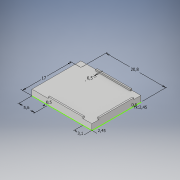
# Autodesk Inventor part: čip
Saved by Autodesk Inventor 2019 (Build 230136000, 136)
## iProperties
Created: 2020-07-28
Part Number: čip
Material: Generic
Document SubType Name: Modeling
Designer: lukad
Density: 1 g/cm^3
Appearance: Default
Author: lukad
Autodesk Inventor part; units mm, degrees
ref_plane "YZ Plane" through (0, 0, 0) normal (1, 0, 0) x (0, 1, 0)
ref_plane "XZ Plane" through (0, 0, 0) normal (0, 1, 0) x (-1, 0, 0)
ref_plane "XY Plane" through (0, 0, 0) normal (0, 0, 1) x (1, 0, 0)
sketch "Sketch1" plane through (0, 0, 0) normal (0, 1, 0) x (-1, 0, 0)
  line L0 (12.4664, 17.9083) -> (-8.3336, 17.9083)
  line L1 (-8.3336, 17.9083) -> (-8.3336, 0.9083)
  line L2 (-8.3336, 0.9083) -> (12.4664, 0.9083)
  line L3 (12.4664, 0.9083) -> (12.4664, 17.9083)
  line L4 (-8.3336, 15.4583) -> (-7.8336, 15.4583)
  line L5 (-7.8336, 15.4583) -> (-7.8336, 3.3583)
  line L6 (-7.8336, 3.3583) -> (-8.3336, 3.3583)
  line L7 (-8.3336, 3.3583) -> (-8.3336, 15.4583)
  line L8 (6.8664, 17.9083) -> (-5.2336, 17.9083)
  line L9 (-5.2336, 17.9083) -> (-5.2336, 17.4083)
  line L10 (-5.2336, 17.4083) -> (6.8664, 17.4083)
  line L11 (6.8664, 17.4083) -> (6.8664, 17.9083)
  line L12 (6.8664, 0.9083) -> (-5.2336, 0.9083)
  line L13 (-5.2336, 0.9083) -> (-5.2336, 1.4083)
  line L14 (-5.2336, 1.4083) -> (6.8664, 1.4083)
  line L15 (6.8664, 1.4083) -> (6.8664, 0.9083)
  point P0 (0, 0)
  dimension "d0" = 20.8
  dimension "d1" = 17
  dimension "d2" = 0.5
  dimension "d3" = 2.45
  dimension "d4" = 2.45
  dimension "d5" = 3.1
  dimension "d6" = 5.6
  dimension "d7" = 0.5
  dimension "d8" = 0.5
  constraints: 32 end point, 8 parallel, 4 horizontal, 4 perpendicular, 3 point on line
  measures "d0" distance between parallel lines of L1 L3
  measures "d1" distance between parallel lines of L2 L0
  measures "d2" distance between parallel lines of L5 L1
  measures "d3" distance between parallel lines of L0 L4
  measures "d4" distance between parallel lines of L2 L6
  measures "d5" distance between parallel lines of L1 L9
  measures "d6" distance between parallel lines of L3 L11
  measures "d7" distance between parallel lines of L10 L0
  measures "d8" distance between parallel lines of L12 L14
extrude "Extrusion1" add sketch "Sketch1" along normal blind 2 contours L3 L2 L15 L14 L13 L1 L6 L5 L4 L0 L9 L10 L11
extrude "Extrusion2" add sketch "Sketch1" along normal blind 2.5 contours L11 L10 L9 L0
extrude "Extrusion3" add sketch "Sketch1" along normal blind 2.5 contours L4 L5 L6 L1
extrude "Extrusion4" add sketch "Sketch1" along normal blind 2.5 contours L2 L13 L14 L15
equation "\"d4\" = d3"
body "Solid1"
